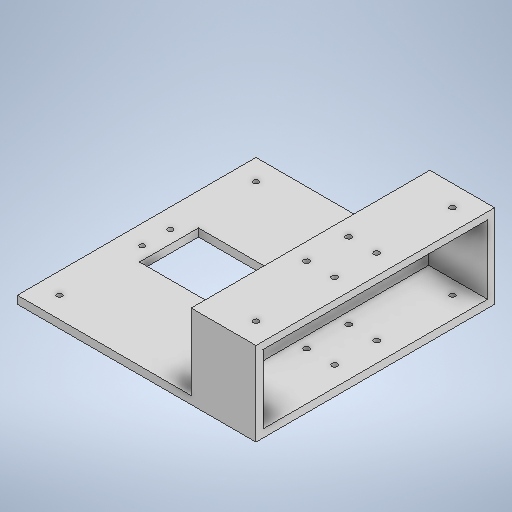
# Autodesk Inventor part: LowerHead
Saved by Autodesk Inventor 2025 (Build 290162000, 162)
## iProperties
Created: 2025-09-02
Part Number: LowerHead
Material: Generic
Document SubType Name: Modeling
Designer: wangb
Density: 1 g/cm^3
Appearance: Default
Author: wangb
Autodesk Inventor part; units mm, degrees
ref_plane "YZ Plane" through (0, 0, 0) normal (1, 0, 0) x (0, 1, 0)
ref_plane "XZ Plane" through (0, 0, 0) normal (0, 1, 0) x (-1, 0, 0)
ref_plane "XY Plane" through (0, 0, 0) normal (0, 0, 1) x (1, 0, 0)
sketch "Sketch1" plane through (0, 0, 0) normal (0, 1, 0) x (-1, 0, 0)
  line L0 (-7.3056, 10.788) -> (-92.3056, 10.788)
  line L1 (-92.3056, 10.788) -> (-92.3056, -74.212)
  line L2 (-92.3056, -74.212) -> (-7.3056, -74.212)
  line L3 (-7.3056, -74.212) -> (-7.3056, 10.788)
  line L4 (-18.8056, -21.212) -> (-59.8056, -21.212)
  line L5 (-59.8056, -21.212) -> (-59.8056, -42.212)
  line L6 (-59.8056, -42.212) -> (-18.8056, -42.212)
  line L7 (-18.8056, -42.212) -> (-18.8056, -21.212)
  circle A0 centre (-14.3056, -26.712) radius 0.9
  circle A1 centre (-14.3056, -36.712) radius 0.9
  circle A2 centre (-64.3056, -26.712) radius 0.9
  circle A3 centre (-64.3056, -36.712) radius 0.9
  circle A4 centre (-14.8056, 3.288) radius 0.95
  circle A5 centre (-84.8056, 3.288) radius 0.95
  circle A6 centre (-14.8056, -66.712) radius 0.95
  circle A7 centre (-84.8056, -66.712) radius 0.95
  circle A8 centre (-75.3056, -39.212) radius 1
  circle A9 centre (-85.3056, -39.212) radius 1
  circle A10 centre (-75.3056, -24.212) radius 1
  circle A11 centre (-85.3052, -24.1286) radius 1
  point P0 (0, 0)
  dimension "d0" = 85
  dimension "d1" = 85
  dimension "d2" = 41
  dimension "d3" = 21
  dimension "d4" = 32
  dimension "d5" = 11.5
  dimension "d6" = 1.8
  dimension "d7" = 1.8
  dimension "d8" = 10
  dimension "d9" = 5.5
  dimension "d10" = 5.5
  dimension "d11" = 1.8
  dimension "d12" = 1.8
  dimension "d13" = 10
  dimension "d14" = 5.5
  dimension "d15" = 50
  dimension "d16" = 50
  dimension "d17" = 4.5
  dimension "d18" = 1.9
  dimension "d19" = 1.9
  dimension "d20" = 1.9
  dimension "d21" = 1.9
  dimension "d22" = 70
  dimension "d23" = 70
  dimension "d24" = 70
  dimension "d25" = 70
  dimension "d26" = 7.5
  dimension "d27" = 7.5
  dimension "d28" = 7.5
  dimension "d31" = 2
  dimension "d32" = 2
  dimension "d33" = 10
  dimension "d34" = 2
  dimension "d35" = 2
  dimension "d36" = 10
  dimension "d37" = 15
  dimension "d38" = 35
  dimension "d39" = 17
  dimension "d40" = 17
  constraints: 16 end point, 12 centre point, 4 parallel, 2 horizontal, 2 perpendicular
  measures "d0" distance of L2.end L1.end
  measures "d1" distance of L1.end L0.end
  measures "d2" distance of L6.end L5.end
  measures "d3" distance of L5.end L4.end
  measures "d4" distance between parallel lines of L2 L6
  measures "d5" distance between parallel lines of L3 L7
  measures "d6" diameter of A0
  measures "d7" diameter of A1
  measures "d8" distance of A1.centre A0.centre
  measures "d9" vertical distance of L4.start A0.centre
  measures "d10" vertical distance of L6.end A1.centre
  measures "d11" diameter of A2
  measures "d12" diameter of A3
  measures "d13" distance of A3.centre A2.centre
  measures "d14" vertical distance of L5.end A3.centre
  measures "d15" distance of A2.centre A0.centre
  measures "d16" distance of A3.centre A1.centre
  measures "d17" distance from line of L5 A2.centre
  measures "d18" diameter of A4
  measures "d19" diameter of A5
  measures "d20" diameter of A6
  measures "d21" diameter of A7
  measures "d22" distance of A5.centre A4.centre
  measures "d23" distance of A7.centre A5.centre
  measures "d24" distance of A6.centre A7.centre
  measures "d25" distance of A6.centre A4.centre
  measures "d26" distance from line of L1 A5.centre
  measures "d27" distance from line of L0 A4.centre
  measures "d28" distance from line of L0 A5.centre
  measures "d31" diameter of A8
  measures "d32" diameter of A9
  measures "d33" distance of A9.centre A8.centre
  measures "d34" diameter of A10
  measures "d35" diameter of A11
  measures "d36" distance of A11.centre A10.centre
  measures "d37" distance of A10.centre A8.centre
  measures "d38" distance from line of L2 A8.centre
  measures "d39" distance from line of A10.centre L1
  measures "d40" distance from line of L1 A8.centre
extrude "Extrusion1" add sketch "Sketch1" along normal blind 2.8 contours L3 L2 L1 L0 | A8 | A9 | A10 | A11
sketch "Sketch2" plane through (0, 2.8, 0) normal (0, 1, 0) x (1, 0, 0)
  circle A0 centre (85.3056, 24.212) radius 1
  circle A1 centre (75.3056, 24.212) radius 1
  circle A2 centre (85.3056, 39.212) radius 1
  circle A3 centre (75.3056, 39.212) radius 1
  line L0 (92.3056, -10.788) -> (92.3056, 74.212) projected
  line L1 (92.3056, 74.212) -> (7.3056, 74.212) projected
  line L2 (7.3056, -10.788) -> (92.3056, -10.788) projected
  point P0 (0, 0)
  dimension "d41" = 2
  dimension "d42" = 2
  dimension "d43" = 10
  dimension "d44" = 2
  dimension "d45" = 2
  dimension "d46" = 10
  dimension "d47" = 15
  dimension "d48" = 7
  dimension "d49" = 35
  dimension "d50" = 35
  dimension "d51" = 35
  dimension "d52" = 35
  constraints: 4 centre point
  measures "d41" diameter of A0
  measures "d42" diameter of A1
  measures "d43" distance of A1.centre A0.centre
  measures "d44" diameter of A2
  measures "d45" diameter of A3
  measures "d46" distance of A3.centre A2.centre
  measures "d47" distance of A2.centre A0.centre
  measures "d48" distance from line of L0 A2.centre
  measures "d49" distance from line of L1 A2.centre
  measures "d50" distance from line of L1 A3.centre
  measures "d51" distance from line of L2 A1.centre
  measures "d52" distance from line of L2 A0.centre
extrude "Extrusion2" cut sketch "Sketch2" against normal blind 50
sketch "Sketch3" plane through (0, 2.8, 0) normal (0, 1, 0) x (1, 0, 0)
  line L0 (7.3056, -10.788) -> (92.3056, -10.788) projected
  line L1 (92.3056, 74.212) -> (7.3056, 74.212) projected
  line L2 (92.3056, -10.788) -> (69.2056, -10.788)
  line L3 (69.2056, -10.788) -> (69.2056, 74.212)
  line L4 (69.2056, 74.212) -> (92.3056, 74.212)
  line L5 (92.3056, 74.212) -> (92.3056, -10.788)
  circle A0 centre (64.3056, 36.712) radius 0.9 projected
  circle A1 centre (75.3056, 24.212) radius 1 projected
  circle A2 centre (75.3056, 24.212) radius 1
  circle A3 centre (75.3056, 39.212) radius 1 projected
  circle A4 centre (75.3056, 39.212) radius 1
  circle A5 centre (85.3056, 39.212) radius 1 projected
  circle A6 centre (85.3056, 39.212) radius 1
  circle A7 centre (85.3056, 24.212) radius 1 projected
  circle A8 centre (85.3056, 24.212) radius 1
  circle A9 centre (84.8056, 66.712) radius 0.95 projected
  circle A10 centre (84.8056, 66.712) radius 1
  circle A11 centre (84.8056, -3.288) radius 0.95 projected
  circle A12 centre (84.8056, -3.288) radius 1
  point P0 (0, 0)
  dimension "d55" = 4
  dimension "d56" = 2
  dimension "d57" = 2
  constraints: 8 end point, 6 centre point, 6 coincident, 2 parallel, 1 horizontal, 1 perpendicular, 1 point on line
  measures "d55" distance edge to line of A0 L3
  measures "d56" diameter of A10
  measures "d57" diameter of A12
extrude "Extrusion3" add sketch "Sketch3" along normal blind 27 contours L3 L1 L5 L0
sketch "Sketch4" plane through (92.3056, 0, 10.788) normal (1, 0, 0) x (0, 0, -1)
  line L0 (85, 2.8) -> (0, 2.8) projected
  line L1 (2.5, 27.3) -> (82.5, 27.3)
  line L2 (82.5, 27.3) -> (82.5, 2.8)
  line L3 (82.5, 2.8) -> (2.5, 2.8)
  line L4 (2.5, 2.8) -> (2.5, 27.3)
  line L5 (0, 0) -> (0, 29.8) projected
  line L6 (85, 0) -> (85, 29.8) projected
  line L7 (0, 0) -> (85, 0) projected
  line L8 (0, 29.8) -> (85, 29.8) projected
  point P0 (10.788, 0)
  point P1 (2.5, 2.8)
  dimension "d60" = 2.5
  dimension "d61" = 2.5
  dimension "d62" = 2.8
  dimension "d63" = 2.5
  constraints: 8 end point, 2 parallel, 1 horizontal, 1 perpendicular, 1 point on line
  measures "d60" distance between parallel lines of L5 L4
  measures "d61" distance between parallel lines of L6 L2
  measures "d62" distance between parallel lines of L7 L0
  measures "d63" distance between parallel lines of L8 L1
extrude "Extrusion4" cut sketch "Sketch4" against normal blind 21 contours L0 L4 L1 L2
body "Solid1"
